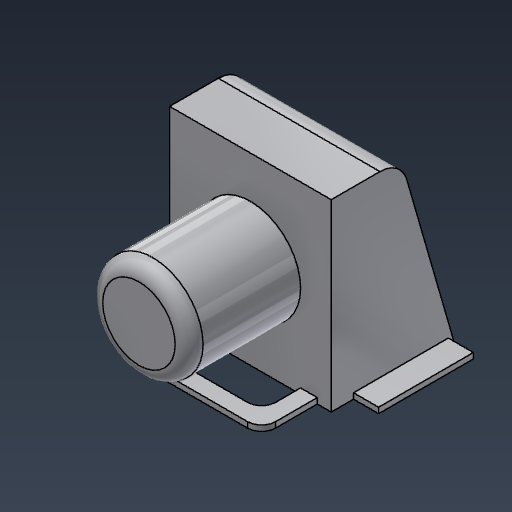
# Autodesk Inventor part: KT11P4
Saved by Autodesk Inventor 2023.1 (Build 271208000, 208)
## iProperties
Created: 2015-08-01
Part Number: KT11P4
Material: PC/ABS-Kunststoff
Document SubType Name: Modeling
Designer: rYan
Mass: 0.062067 g
Surface Area: 2.29622 cm^2
Volume: 0.173725 cm^3
Density: 0.357273 g/cm^3
Appearance: Glatt - weiß
Author: rYan
Autodesk Inventor part; units mm, degrees
ref_plane "YZ Plane" through (0, 0, 0) normal (1, 0, 0) x (0, 1, 0)
ref_plane "XZ Plane" through (0, 0, 0) normal (0, 1, 0) x (-1, 0, 0)
ref_plane "XY Plane" through (0, 0, 0) normal (0, 0, 1) x (1, 0, 0)
sketch "Skizze2" plane through (0, 0, 0) normal (1, 0, 0) x (0, 1, 0)
  line L0 (0, 0) -> (4.4, 0)
  line L1 (2.5, 6.6) -> (0, 6.6)
  line L2 (0, 6.6) -> (0, 0)
  line L3 (2.5, 6.6) -> (4.4, 0)
  line L4 (-0.88, 0) -> (5.28, 0) projected
  line L5 (0, 7.92) -> (0, -1.32) projected
  dimension "d2" = 6.6
  dimension "d3" = 2.5
  dimension "d4" = 4.4
  constraints: 8 end point, 1 collinear, 1 horizontal, 1 parallel
  measures "d2" distance of L1.end L0.start
  measures "d3" distance of L1.start L1.end
  measures "d4" distance of L0.start L0.end
extrude "Extrusion1" add sketch "Skizze2" along normal mid plane 5.8
sketch "Skizze3" plane through (-2.9, 0, 0) normal (0, -1, 0) x (1, 0, 0)
  line L0 (5.8, 0) -> (0, 0) projected
  line L1 (5.8, 6.6) -> (5.8, 0) projected
  line L2 (0, 6.6) -> (5.8, 6.6) projected
  line L3 (0, 0) -> (0, 6.6) projected
  line L4 (0, 6.6) -> (0, 0) construction
  line L5 (0, 3.3) -> (5.8, 3.3) construction
  line L6 (5.8, 0) -> (5.8, 6.6) construction
  line L7 (0, 6.6) -> (5.8, 6.6) construction
  line L8 (2.9, 6.6) -> (2.9, 0) construction
  circle A0 centre (2.9, 3.3) radius 1.8
  dimension "d7" = 3.6
  constraints: 4 end point, 4 midpoint, 1 centre point, 1 vertical
  measures "d7" diameter of A0
extrude "Extrusion2" add sketch "Skizze3" along normal blind 4 contours A0
sketch "Skizze4" plane through (2.9, 4.4, 0) normal (0, 0, -1) x (-1, 0, 0)
  line L0 (5.8, 0) -> (0, 0) projected
  line L1 (0, -4.4) -> (0, 0) projected
  line L2 (0, -4.4) -> (5.8, -4.4) projected
  line L3 (5.8, 0) -> (5.8, -4.4) projected
  line L4 (0, -4.4) -> (0, 0) projected
  line L5 (0, -3.6) -> (-0.9, -3.6)
  line L6 (-0.9, -3.6) -> (-0.9, -0.2)
  line L7 (-0.9, -0.2) -> (0, -0.2)
  line L8 (0, -0.2) -> (0, -3.6)
  line L9 (5.8, -4.4) -> (0, -4.4) projected
  line L10 (5.3, -4.4) -> (5.3, -6.4)
  line L11 (5.3, -6.4) -> (0.5, -6.4)
  line L12 (0.5, -6.4) -> (0.5, -4.4)
  line L13 (2.9, -4.4) -> (2.9, 0) construction
  line L14 (5.8, 0) -> (0, 0) construction
  line L15 (4.7, -4.4) -> (4.7, -5.8)
  line L16 (4.7, -5.8) -> (1.1, -5.8)
  line L17 (1.1, -5.8) -> (1.1, -4.4)
  line L18 (0.5, -4.4) -> (1.1, -4.4)
  line L19 (4.7, -4.4) -> (5.3, -4.4)
  line L20 (0, -4.4) -> (5.8, -4.4) projected
  line L21 (5.8, -1.9) -> (5.8, 0) projected
  line L22 (5.8, -0.2) -> (6.7, -0.2)
  line L23 (6.7, -0.2) -> (6.7, -3.6)
  line L24 (6.7, -3.6) -> (5.8, -3.6)
  line L25 (5.8, -3.6) -> (5.8, -0.2)
  dimension "d10" = 0.8
  dimension "d11" = 3.4
  dimension "d12" = 0.9
  dimension "d13" = 2
  dimension "d14" = 4.8
  dimension "d16" = 0.6
  dimension "d17" = 0.6
  dimension "d18" = 0.9
  constraints: 34 end point, 9 parallel, 4 horizontal, 4 perpendicular, 3 point on line, 1 collinear, 1 midpoint, 4 other
  measures "d10" distance between parallel lines of L5 L2
  measures "d11" distance of L5.end L6.end
  measures "d12" distance of L6.end L7.end
  measures "d13" distance of L11.end L12.end
  measures "d14" distance of L10.end L11.end
  measures "d16" distance between parallel lines of L11 L16
  measures "d17" distance between parallel lines of L12 L17
  measures "d18" distance of L22.start L22.end
extrude "Extrusion3" add sketch "Skizze4" against normal blind 0.2 contours L22 L23 L24 L3 | L1 L5 L6 L7 | L2 L17 L16 L15 L10 L11 L12
fillet "Rundung1" radius 1 1 edges at (0, 2.5, 6.6)
fillet "Rundung2" radius 0.5 1 edges at (-1.8, -4, 3.3)
fillet "Rundung3" radius 0.5 4 edges at (-2.4, -2, 0.1) (2.4, -2, 0.1) (1.8, -1.4, 0.1) (-1.8, -1.4, 0.1)
equation "\"d17\" = d16"
equation "\"d18\" = d12"
